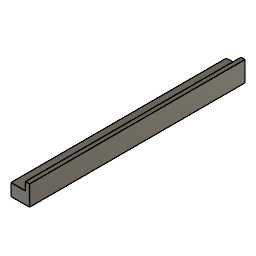
cover rolls mount left part 2 (Autodesk Fusion 360 design; units mm, degrees)
Autodesk Fusion 360 part; units mm, degrees
sketch "Szkic1" plane through (0, 0, 0) normal (0, 0, 1) x (1, 0, 0)
  line L0 (-35, 125) -> (-35, -140)
  line L1 (-35, -140) -> (45, -140)
  line L2 (45, 125) -> (-35, 125)
  circle A0 centre (-25, 115) radius 1.75
  circle A1 centre (25, 115) radius 1.75
  circle A2 centre (-25, 65) radius 1.75
  circle A3 centre (-25, 15) radius 1.75
  circle A4 centre (-25, -35) radius 1.75
  circle A5 centre (-25, -85) radius 1.75
  circle A6 centre (-15, -110) radius 3.5
  circle A7 centre (-15, -130) radius 3.5
  circle A8 centre (20, -130) radius 3.5
  circle A9 centre (20, -110) radius 3.5
  line L3 (-35, 125) -> (-35, 100)
  line L4 (-35, 100) -> (45, 100)
  line L5 (45, 100) -> (45, 125)
  line L6 (45, 125) -> (-35, 125)
  line L7 (-35, -140) -> (-17, -140)
  line L8 (-17, -140) -> (-17, 100)
  line L9 (-17, 100) -> (-35, 100)
  line L10 (-35, 100) -> (-35, -140)
  line L11 (-17, -140) -> (-17, 100)
  line L12 (-17, 100) -> (-12, 100)
  line L13 (-12, 100) -> (-12, -140)
  line L14 (-12, -140) -> (-17, -140)
  dimension "d1" = 18
  dimension "d2" = 5
  constraint perpendicular L3 L4
  constraint parallel L3 L5
  constraint parallel L4 L6
  constraint coincident L0 L3.end
  constraint perpendicular L2 L3
  constraint perpendicular L7 L8
  constraint parallel L7 L9
  constraint parallel L8 L10
  constraint perpendicular L0 L7
  constraint perpendicular L11 L12
  constraint parallel L11 L13
  constraint parallel L12 L14
  measures "d1" distance of L0.end L7.end
  measures "d2" distance of L7.end L13.end
extrude "Wyciągnięcie proste1" add sketch "Szkic1" along normal blind 15 contours L0 L1 A6 A7 L4 L7 L8 L9 L10 L11 | A6 L8 L11 | A7 L8 L11
extrude "Wyciągnięcie proste2" add sketch "Szkic1" along normal blind 25 contours A6 L4 L8 L11 L12 L13 | L1 A7 L8 L11 L13 L14 | A6 L8 L11 L13 | A7 L8 L11 L13 | A6 A7 L8 L11 L13
extrude "Wyciągnięcie proste3" add 1 faces at (-21.3333, 100, 5) along direction (0, 1, 0) blind 26
extrude "Wyciągnięcie proste4" cut sketch "Szkic1" along normal blind 42 contours A0
sketch "Szkic2" plane through (0, 0, 0) normal (0, 0, -1) x (1, 0, 0)
  circle A0 centre (-25, -115) radius 1.75
  circle A1 centre (-25, -65) radius 1.75
  circle A2 centre (-25, -15) radius 1.75
  circle A3 centre (-25, 35) radius 1.75
  circle A4 centre (-25, 85) radius 1.75
  line L0 (-12, 140) -> (-35, 140)
  line L1 (-35, 140) -> (-35, -126)
  line L2 (-35, -126) -> (-12, -126)
  line L3 (-12, -126) -> (-12, 140)
  circle A5 centre (-25, 85) radius 2
  circle A6 centre (-25, 35) radius 2
  circle A7 centre (-25, -15) radius 2
  circle A8 centre (-25, -65) radius 2
  circle A9 centre (-25, -115) radius 2
  circle A10 centre (-25, -115) radius 3.5
  dimension "d11" = 4
  dimension "d12" = 4
  dimension "d13" = 4
  dimension "d14" = 4
  dimension "d15" = 4
  dimension "d16" = 7
  constraint concentric A4 A5
  constraint concentric A3 A6
  constraint concentric A2 A7
  constraint concentric A1 A8
  constraint concentric A0 A9
  constraint concentric A9 A10
  measures "d11" diameter of A5
  measures "d12" diameter of A6
  measures "d13" diameter of A7
  measures "d14" diameter of A8
  measures "d15" diameter of A9
  measures "d16" diameter of A10
extrude "Wyciągnięcie proste5" cut sketch "Szkic2" against normal blind 100 contours A5 | A6 | A7 | A8 | A9
extrude "Wyciągnięcie proste6" cut sketch "Szkic2" against normal blind 4 contours A10
